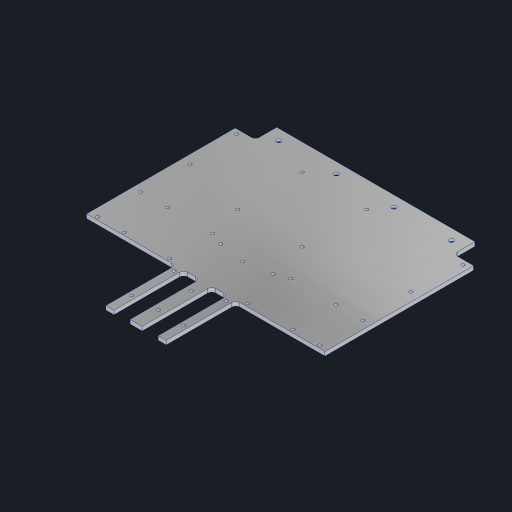
# Autodesk Inventor part: base
Saved by Autodesk Inventor 2023 (Build 270158000, 158)
## iProperties
Created: 2024-04-10
Part Number: base
Material: Aluminum 6061
Document SubType Name: Modeling
Designer: szymo
Density: 2.7 g/cm^3
Appearance: Aluminum - Flat
Mass: 138.037 g
Surface Area: 408.524 cm^2
Volume: 51.1249 cm^3
Author: szymo
Autodesk Inventor part; units mm, degrees
ref_plane "YZ Plane" through (0, 0, 0) normal (1, 0, 0) x (0, 1, 0)
ref_plane "XZ Plane" through (0, 0, 0) normal (0, 1, 0) x (-1, 0, 0)
ref_plane "XY Plane" through (0, 0, 0) normal (0, 0, 1) x (1, 0, 0)
sketch "Sketch2" plane through (0, 0, 0) normal (0, 1, 0) x (-1, 0, 0)
  line L0 (-89, 99) -> (89, 99)
  line L1 (89, 99) -> (89, -99)
  line L2 (89, -99) -> (-89, -99)
  line L3 (-89, -99) -> (-89, 99)
  line L4 (-89, 99) -> (89, -99) construction
  line L5 (89, 99) -> (-89, -99) construction
  line L6 (-89, 99) -> (89, 99)
  line L7 (89, 99) -> (89, -81)
  line L8 (89, -81) -> (-89, -81)
  line L9 (-89, -81) -> (-89, 99)
  line L10 (-4.5, 99) -> (-89, 99)
  line L11 (-89, 99) -> (-89, 46)
  line L12 (-89, 46) -> (-4.5, 46)
  line L13 (-4.5, 46) -> (-4.5, 99)
  line L14 (4.5, 99) -> (89, 99)
  line L15 (89, 99) -> (89, 46)
  line L16 (89, 46) -> (4.5, 46)
  line L17 (4.5, 46) -> (4.5, 99)
  line L18 (22.5, 77.5) -> (22.5, 66.5) projected
  line L19 (16.5, 66.5) -> (16.5, 77.5) projected
  line L20 (-22.5, 66.5) -> (-22.5, 77.5) projected
  line L21 (-16.5, 77.5) -> (-16.5, 66.5) projected
  line L22 (-22.5, 99) -> (-16.5, 99)
  line L23 (-16.5, 99) -> (-16.5, 46)
  line L24 (-16.5, 46) -> (-22.5, 46)
  line L25 (-22.5, 46) -> (-22.5, 99)
  line L26 (16.5, 99) -> (22.5, 99)
  line L27 (22.5, 99) -> (22.5, 46)
  line L28 (22.5, 46) -> (16.5, 46)
  line L29 (16.5, 46) -> (16.5, 99)
  line L30 (-89, 99) -> (89, 99)
  line L31 (89, 99) -> (89, 98)
  line L32 (89, 98) -> (-89, 98)
  line L33 (-89, 98) -> (-89, 99)
  line L34 (89, -81) -> (74, -81)
  line L35 (74, -81) -> (74, -65)
  line L36 (74, -65) -> (89, -65)
  line L37 (89, -65) -> (89, -81)
  line L38 (-89, -81) -> (-74, -81)
  line L39 (-74, -81) -> (-74, -65)
  line L40 (-74, -65) -> (-89, -65)
  line L41 (-89, -65) -> (-89, -81)
  point P0 (0, 0)
  point P1 (4.5, 99)
  point P2 (-4.5, 99)
  point P3 (-89, 46)
  point P4 (89, 46)
  point P5 (4.5, 98)
  point P6 (-4.5, 98)
  point P7 (-16.5, 98)
  point P8 (-22.5, 98)
  point P9 (22.5, 98)
  point P10 (16.5, 98)
  dimension "d8" = 178
  dimension "d9" = 198
  dimension "d10" = 18
  dimension "d11" = 84.5
  dimension "d12" = 53
  dimension "d13" = 84.5
  dimension "d14" = 53
  dimension "d17" = 9
  dimension "d18" = 1
  dimension "d19" = 15
  dimension "d20" = 16
  dimension "d21" = 15
  dimension "d22" = 16
  constraints: 76 end point, 18 parallel, 9 horizontal, 9 perpendicular, 7 point on line, 4 collinear, 2 midpoint, 5 other
  measures "d8" distance of L1.end L2.end
  measures "d9" distance of L0.end L1.end
  measures "d10" distance between parallel lines of L8 L2
  measures "d11" distance of L12.end L11.end
  measures "d12" distance of L0.start L11.end
  measures "d13" distance of L15.end L16.end
  measures "d14" distance of L6.end L15.end
  measures "d17" distance between parallel lines of L13 L17
  measures "d18" distance of L30.end L31.end
  measures "d19" distance of L35.end L36.end
  measures "d20" distance of L34.end L35.end
  measures "d21" distance of L40.end L39.end
  measures "d22" distance of L39.end L38.end
extrude "Extrusion2" add sketch "Sketch2" along normal blind 3 contours L32 L23 L21 L12 L25 L20 | L12 L13 L32 L17 L16 L1 L36 L35 L8 L39 L40 L3 | L32 L27 L18 L16 L29 L19
sketch "Sketch3" plane through (0, 0, 0) normal (0, -1, 0) x (1, 0, 0)
  circle A0 centre (19.5, 81.925) radius 1.8 projected
  circle A1 centre (0, 81.3875) radius 1.8 projected
  circle A2 centre (-19.5, 81.925) radius 1.8 projected
  circle A3 centre (-19.5, 50.2091) radius 1.8 projected
  circle A4 centre (0, 56.4774) radius 1.8 projected
  circle A5 centre (19.5, 50.2091) radius 1.8 projected
  circle A6 centre (62.9, 43.8) radius 1.8 projected
  circle A7 centre (83, 43.8) radius 1.8 projected
  circle A8 centre (83, 11.6615) radius 1.8 projected
  circle A9 centre (62.9, 11.6615) radius 1.8 projected
  circle A10 centre (29.2, 11.6615) radius 1.8 projected
  circle A11 centre (29.2, 43.8) radius 1.8 projected
  circle A12 centre (19.5, 15.3216) radius 1.8 projected
  circle A13 centre (19.5, 50.2091) radius 1.8 projected
  circle A14 centre (0, 56.4774) radius 1.8 projected
  circle A15 centre (0, 18.5615) radius 1.8 projected
  circle A16 centre (-19.5, 15.3216) radius 1.8 projected
  circle A17 centre (-19.5, 50.2091) radius 1.8 projected
  circle A18 centre (-29.2, 43.8) radius 1.8 projected
  circle A19 centre (-29.2, 11.6615) radius 1.8 projected
  circle A20 centre (-62.9, 11.6615) radius 1.8 projected
  circle A21 centre (-62.9, 43.8) radius 1.8 projected
  circle A22 centre (-83, 43.8) radius 1.8 projected
  circle A23 centre (-83, 11.6615) radius 1.8 projected
  circle A24 centre (-82.5, -24.6725) radius 1.8 projected
  circle A25 centre (-35.4342, -13.2005) radius 1.6 projected
  circle A26 centre (-35.4342, -61.4005) radius 1.6 projected
  circle A27 centre (12.7658, -61.4005) radius 1.6 projected
  circle A28 centre (12.7658, -13.2005) radius 1.6 projected
  circle A29 centre (82.5, -24.6725) radius 1.8 projected
  circle A30 centre (84.5, -61.5) radius 1.8 projected
  circle A31 centre (-84.5, -61.5) radius 1.8 projected
  circle A32 centre (-66, -77) radius 1.8 projected
  circle A33 centre (-22, -77) radius 1.8 projected
  circle A34 centre (22, -77) radius 1.8 projected
  circle A35 centre (66, -77) radius 1.8 projected
  point P0 (0, 0)
  constraints: 29 coincident
hole "Hole1" at (-19.5, 0, 81.925) at (0, 0, 81.3875) at (19.5, 0, 81.925) at (19.5, 0, 50.2091) at (0, 0, 56.4774) at (-19.5, 0, 50.2091) at (-83, 0, 43.8) at (-62.9, 0, 43.8) at (-29.2, 0, 43.8) at (29.2, 0, 43.8) at (62.9, 0, 43.8) at (83, 0, 43.8) at (83, 0, 11.6615) at (62.9, 0, 11.6615) at (29.2, 0, 11.6615) at (19.5, 0, 15.3216) at (0, 0, 18.5615) at (-19.5, 0, 15.3216) at (-29.2, 0, 11.6615) at (-62.9, 0, 11.6615) at (-83, 0, 11.6615) at (82.5, 0, -24.6725) at (12.7658, 0, -13.2005) at (-35.4342, 0, -13.2005) at (-82.5, 0, -24.6725) at (-84.5, 0, -61.5) at (-35.4342, 0, -61.4005) at (12.7658, 0, -61.4005) at (84.5, 0, -61.5) direction (0, 1, 0) diameter 2.459 end through all thread size "M3x0.5" class "6H" standard "ANSI Metric M Profile"
fillet "Fillet1" radius 3 6 edges at (22.5, 1.5, 46) (-22.5, 1.5, 46) (-16.5, 1.5, 46) (-4.5, 1.5, 46) (4.5, 1.5, 46) (16.5, 1.5, 46)
fillet "Fillet2" radius 3 2 edges at (74, 1.5, -65) (-74, 1.5, -65)
sketch "Sketch5" plane through (0, 0, 0) normal (0, -1, 0) x (1, 0, 0)
  circle A0 centre (64.5, -73) radius 1.2295 projected
  circle A1 centre (21.5, -73) radius 1.2295 projected
  circle A2 centre (-21.5, -73) radius 1.2295 projected
  circle A3 centre (-64.5, -73) radius 1.2295 projected
  point P0 (0, 0)
hole "Hole2" at (64.5, 0, -73) at (21.5, 0, -73) at (-21.5, 0, -73) at (-64.5, 0, -73) direction (0, 1, 0) diameter 3.6 end through all countersink diameter 6.5 countersink angle 90 clearance for "Countersunk Flat Head Screw ISO 2009/7046" size "M3" standard "ISO"
equation "\"d11\" = d13"
body "Solid2"
